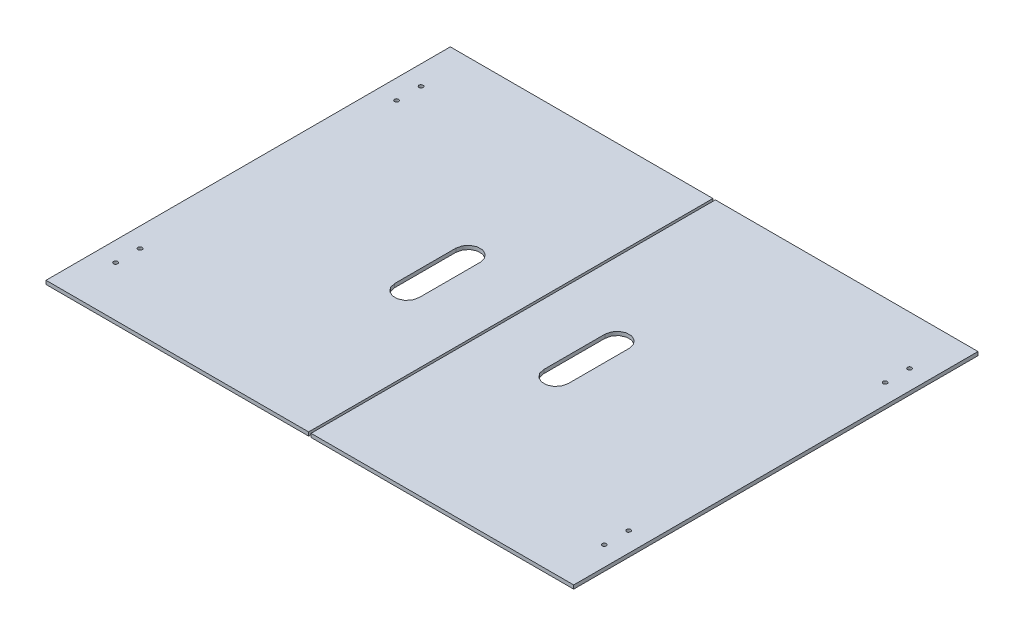
# Autodesk Inventor part: Door Panel
Saved by Autodesk Inventor 2023.2 (Build 272271000, 271)
## iProperties
Created: 2023-03-05
Part Number: Door Panel
Material: PMMA Plastic
Document SubType Name: Modeling
Designer: remop
Density: 1.188 g/cm^3
Appearance: Polycarbonate - Clear
Author: remop
Autodesk Inventor part; units mm, degrees
ref_plane "YZ Plane" through (0, 0, 0) normal (1, 0, 0) x (0, 1, 0)
ref_plane "XZ Plane" through (0, 0, 0) normal (0, 1, 0) x (-1, 0, 0)
ref_plane "XY Plane" through (0, 0, 0) normal (0, 0, 1) x (1, 0, 0)
sketch "Sketch1" plane through (0, 0, 0) normal (0, 1, 0) x (-1, 0, 0)
  circle A0 centre (104.8829, 126.4348) radius 1.25 projected
  circle A1 centre (139.8829, 126.4348) radius 1.25 projected
  circle A2 centre (-92.6171, 155.4348) radius 1.6 projected
  circle A3 centre (210.3829, 138.4348) radius 11.5 projected
  circle A4 centre (-92.6171, 114.4348) radius 1.6 projected
  line L0 (-122.7381, 154.8468) -> (-122.7381, 115.0468) projected
  line L1 (-122.7381, 115.0468) -> (-181.8381, 115.0468) projected
  line L2 (-181.8381, 115.0468) -> (-181.8381, 154.8468) projected
  line L3 (-181.8381, 154.8468) -> (-122.7381, 154.8468) projected
  circle A5 centre (95.3829, 138.4348) radius 12.5 projected
  circle A6 centre (130.3829, 138.4348) radius 12.5 projected
  circle A7 centre (120.8829, 150.4348) radius 1.25 projected
  circle A8 centre (-102.5711, 120.4348) radius 2.5 projected
  circle A9 centre (-185.6171, 155.4348) radius 1.6 projected
  circle A10 centre (-185.6171, 114.4348) radius 1.6 projected
  circle A11 centre (-102.5711, 138.2317) radius 4.5 projected
  circle A12 centre (85.8829, 150.4348) radius 1.25 projected
  circle A13 centre (-52.5711, 138.4348) radius 8 projected
  line L4 (240.3829, 518.4348) -> (240.3829, 185.4348) projected
  line L5 (240.3829, 185.4348) -> (-193.6171, 185.4348) projected
  line L6 (-193.6171, 185.4348) -> (-193.6171, 518.4348) projected
  line L7 (-193.6171, 518.4348) -> (240.3829, 518.4348) projected
  line L8 (290.3829, 78.4348) -> (-243.6171, 78.4348) projected
  line L9 (290.3829, 558.4348) -> (290.3829, 78.4348) projected
  line L10 (-243.6171, 558.4348) -> (290.3829, 558.4348) projected
  line L11 (-243.6171, 78.4348) -> (-243.6171, 558.4348) projected
  circle A14 centre (-234.1171, 143.4348) radius 1.75 projected
  circle A15 centre (-141.6171, 550.9348) radius 1.75 projected
  circle A16 centre (23.3829, 550.9348) radius 1.75 projected
  circle A17 centre (188.3829, 85.9348) radius 1.75 projected
  circle A18 centre (23.3829, 85.9348) radius 1.75 projected
  circle A19 centre (-141.6171, 85.9348) radius 1.75 projected
  circle A20 centre (280.8829, 493.4348) radius 1.75 projected
  circle A21 centre (280.8829, 143.4348) radius 1.75 projected
  circle A22 centre (-234.1171, 493.4348) radius 1.75 projected
  circle A23 centre (188.3829, 550.9348) radius 1.75 projected
  circle A24 centre (-176.6171, 226.4348) radius 1.75 projected
  circle A25 centre (-176.6171, 246.4348) radius 1.75 projected
  circle A26 centre (-176.6171, 456.4348) radius 1.75 projected
  circle A27 centre (-176.6171, 476.4348) radius 1.75 projected
  circle A28 centre (223.3829, 476.4348) radius 1.75 projected
  circle A29 centre (223.3829, 456.4348) radius 1.75 projected
  circle A30 centre (223.3829, 226.4348) radius 1.75 projected
  circle A31 centre (223.3828, 246.4348) radius 1.75 projected
  line L12 (-192.6171, 517.4348) -> (239.3829, 517.4348)
  line L13 (239.3829, 517.4348) -> (239.3829, 186.4348)
  line L14 (239.3829, 186.4348) -> (-192.6171, 186.4348)
  line L15 (-192.6171, 186.4348) -> (-192.6171, 517.4348)
  point P0 (0, 0)
  dimension "d0" = 1
  dimension "d1" = 1
  dimension "d2" = 1
  dimension "d3" = 1
  constraints: 8 end point, 2 parallel, 1 horizontal, 1 perpendicular
  measures "d0" distance between parallel lines of L5 L14
  measures "d1" distance between parallel lines of L4 L13
  measures "d2" distance between parallel lines of L7 L12
  measures "d3" distance between parallel lines of L15 L6
extrude "Extrusion1" add sketch "Sketch1" against normal blind 3 contours L12 L13 L14 L15
sketch "Sketch2" plane through (0, 0, 0) normal (0, 1, 0) x (1, 0, 0)
  line L0 (192.6171, -186.4348) -> (-239.3829, -186.4348) projected
  line L1 (-239.3829, -186.4348) -> (-239.3829, -517.4348) projected
  line L2 (-239.3829, -517.4348) -> (192.6171, -517.4348) projected
  line L3 (192.6171, -517.4348) -> (192.6171, -186.4348) projected
  circle A0 centre (176.6171, -476.4348) radius 1.75 projected
  circle A1 centre (176.6171, -246.4348) radius 1.75 projected
  circle A2 centre (176.6171, -226.4348) radius 1.75 projected
  circle A3 centre (176.6171, -456.4348) radius 1.75 projected
  line L4 (-239.3829, -186.4348) -> (192.6171, -186.4348) projected
  line L5 (-22.3829, -186.4348) -> (-22.3829, -517.4348)
  line L6 (192.6171, -517.4348) -> (-239.3829, -517.4348) projected
  line L7 (-24.3829, -517.4348) -> (-24.3829, -186.4348)
  circle A4 centre (-23.3829, -203.4348) radius 3 projected
  line L8 (37.6171, -376.9348) -> (37.6171, -326.9348) construction
  line L9 (27.6171, -376.9348) -> (27.6171, -326.9348)
  line L10 (47.6171, -326.9348) -> (47.6171, -376.9348)
  arc A5 (27.6171, -376.9348) -> (47.6171, -376.9348) centre (37.6171, -376.9348) ccw
  arc A6 (47.6171, -326.9348) -> (27.6171, -326.9348) centre (37.6171, -326.9348) ccw
  line L11 (-84.3829, -376.9348) -> (-84.3829, -326.9348) construction
  line L12 (-74.3829, -376.9348) -> (-74.3829, -326.9348)
  line L13 (-94.3829, -326.9348) -> (-94.3829, -376.9348)
  arc A7 (-94.3829, -376.9348) -> (-74.3829, -376.9348) centre (-84.3829, -376.9348) ccw
  arc A8 (-74.3829, -326.9348) -> (-94.3829, -326.9348) centre (-84.3829, -326.9348) ccw
  point P0 (0, 0)
  point P1 (37.6171, -351.9348)
  point P2 (-84.3829, -351.9348)
  point P3 (-24.3829, -351.9348)
  point P4 (-22.3829, -351.9348)
  point P5 (-22.3829, -206.2632)
  point P6 (-24.3829, -206.2632)
  point P7 (-24.3829, -517.4348)
  dimension "d6" = 1
  dimension "d7" = 1
  dimension "d8" = 50
  dimension "d9" = 50
  dimension "d10" = 50
  dimension "d11" = 10
  constraints: 20 end point, 8 point on circle, 8 tangent, 4 centre point, 4 midpoint, 4 parallel, 4 point on line, 2 horizontal alignment, 2 perpendicular, 1 equal radius, 1 vertical
  measures "d6" distance from line of L7 A4.centre
  measures "d7" distance from line of L5 A4.centre
  measures "d8" distance between parallel lines of L9 L5
  measures "d9" distance between parallel lines of L7 L12
  measures "d10" distance of L9.start L9.end
  measures "d11" radius of A5
extrude "Extrusion2" cut sketch "Sketch2" against normal blind 3 contours L5 A4 L7 L0 | L5 A4 L7 | L2 L7 A4 L5 | L9 A6 L10 A5 | A7 L13 A8 L12
equation "\"d1\" = d0"
equation "\"d2\" = d0"
equation "\"d3\" = d0"
equation "\"d7\" = d6"
equation "\"d9\" = d8"
body "Solid1"
